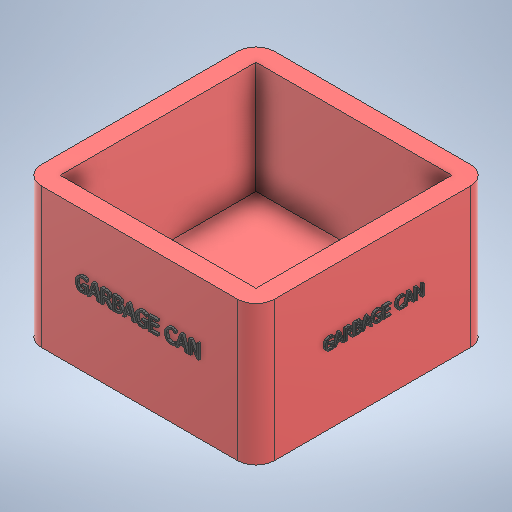
# Autodesk Inventor part: Garbage Can Mockup
Saved by Autodesk Inventor 2025.2 (Build 292293000, 293)
## iProperties
Created: 2025-01-24
Part Number: Garbage Can Mockup
Material: Generic
Document SubType Name: Modeling
Designer: Matt Tidd
Density: 1 g/cm^3
Appearance: Default
Author: Matt Tidd
Autodesk Inventor part; units mm, degrees
ref_plane "YZ Plane" through (0, 0, 0) normal (1, 0, 0) x (0, 1, 0)
ref_plane "XZ Plane" through (0, 0, 0) normal (0, 1, 0) x (-1, 0, 0)
ref_plane "XY Plane" through (0, 0, 0) normal (0, 0, 1) x (1, 0, 0)
sketch "Sketch1" plane through (0, 0, 0) normal (0, 1, 0) x (-1, 0, 0)
  line L0 (0, 0) -> (250, 0)
  line L1 (250, 0) -> (250, -250)
  line L2 (250, -250) -> (0, -250)
  line L3 (0, -250) -> (0, 0)
  dimension "d0" = 250
  dimension "d1" = 250
  constraints: 8 end point, 2 parallel, 1 horizontal, 1 perpendicular
  measures "d0" distance of L1.end L2.end
  measures "d1" distance of L0.end L1.end
extrude "Extrusion1" add sketch "Sketch1" along normal blind 150
fillet "Fillet1" radius 20 4 edges at (0, 75, 0) (-250, 75, 0) (0, 75, -250) (-250, 75, -250)
sketch "Sketch2" plane through (-230, 0, 0) normal (0, 0, 1) x (1, 0, 0)
  line L0 (-20, 0) -> (-20, 150) construction
  line L1 (-20, 75) -> (230, 75) construction
  line L2 (230, 150) -> (230, 0) construction
  spline S0 degree 2 poles (45.9056, 74.7083) (44.3132, 74.7083) (41.6754, 75.6807) (40.7273, 76.6653) knots 0 0 0 1 2 2 2
  spline S1 degree 2 poles (40.7273, 76.6653) (39.7792, 77.6621) (38.7703, 80.6037) (38.7703, 82.5122) knots 0 0 0 1 2 2 2
  spline S2 degree 2 poles (38.7703, 82.5122) (38.7703, 84.3233) (39.7913, 87.1921) (40.7395, 88.2131) knots 0 0 0 1 2 2 2
  spline S3 degree 2 poles (40.7395, 88.2131) (41.6511, 89.1977) (44.3254, 90.2674) (45.9177, 90.2674) knots 0 0 0 1 2 2 2
  spline S4 degree 2 poles (45.9177, 90.2674) (46.6835, 90.2674) (48.0693, 90.0486) (48.7014, 89.8541) knots 0 0 0 1 2 2 2
  spline S5 degree 2 poles (48.7014, 89.8541) (49.2119, 89.7083) (50.4518, 89.1734) (50.8286, 88.9789) knots 0 0 0 1 2 2 2
  line L3 (50.8286, 88.9789) -> (50.8286, 86.5721)
  line L4 (50.8286, 86.5721) -> (50.6584, 86.5721)
  spline S6 degree 2 poles (50.6584, 86.5721) (50.2816, 86.9003) (49.4915, 87.4959) (48.7622, 87.8363) knots 0 0 0 1 2 2 2
  spline S7 degree 2 poles (48.7622, 87.8363) (48.1544, 88.1402) (46.5863, 88.5413) (45.6868, 88.5413) knots 0 0 0 1 2 2 2
  spline S8 degree 2 poles (45.6868, 88.5413) (43.5231, 88.5413) (40.8489, 85.2836) (40.8489, 82.5729) knots 0 0 0 1 2 2 2
  spline S9 degree 2 poles (40.8489, 82.5729) (40.8489, 81.0656) (41.5539, 78.8047) (42.2224, 78.0267) knots 0 0 0 1 2 2 2
  spline S10 degree 2 poles (42.2224, 78.0267) (42.8667, 77.2488) (44.69, 76.4344) (45.8327, 76.4344) knots 0 0 0 1 2 2 2
  spline S11 degree 2 poles (45.8327, 76.4344) (46.6714, 76.4344) (48.3489, 76.6775) (48.9202, 76.9206) knots 0 0 0 1 2 2 2
  line L5 (48.9202, 76.9206) -> (48.9202, 80.7982)
  line L6 (48.9202, 80.7982) -> (45.4437, 80.7982)
  line L7 (45.4437, 80.7982) -> (45.4437, 82.5486)
  line L8 (45.4437, 82.5486) -> (50.8894, 82.5486)
  line L9 (50.8894, 82.5486) -> (50.8894, 75.9968)
  spline S12 degree 2 poles (50.8894, 75.9968) (50.5126, 75.8266) (49.2241, 75.3039) (48.6771, 75.1459) knots 0 0 0 1 2 2 2
  spline S13 degree 2 poles (48.6771, 75.1459) (47.9356, 74.9271) (46.7443, 74.7083) (45.9056, 74.7083) knots 0 0 0 1 2 2 2
  line L10 (51.7767, 75) -> (56.8335, 90)
  line L11 (56.8335, 90) -> (59.2889, 90)
  line L12 (59.2889, 90) -> (64.3456, 75)
  line L13 (64.3456, 75) -> (62.2427, 75)
  line L14 (62.2427, 75) -> (60.8813, 79.1937)
  line L15 (60.8813, 79.1937) -> (55.156, 79.1937)
  line L16 (55.156, 79.1937) -> (53.7946, 75)
  line L17 (53.7946, 75) -> (51.7767, 75)
  line L18 (60.3343, 80.8955) -> (58.0126, 87.9579)
  line L19 (58.0126, 87.9579) -> (55.703, 80.8955)
  line L20 (55.703, 80.8955) -> (60.3343, 80.8955)
  line L21 (77.5709, 75) -> (74.9818, 75)
  line L22 (74.9818, 75) -> (70.2411, 80.9684)
  line L23 (70.2411, 80.9684) -> (67.9558, 80.9684)
  line L24 (67.9558, 80.9684) -> (67.9558, 75)
  line L25 (67.9558, 75) -> (65.9623, 75)
  line L26 (65.9623, 75) -> (65.9623, 90)
  line L27 (65.9623, 90) -> (69.8278, 90)
  spline S14 degree 2 poles (69.8278, 90) (71.1163, 90) (72.8545, 89.7204) (73.6447, 89.2099) knots 0 0 0 1 2 2 2
  spline S15 degree 2 poles (73.6447, 89.2099) (74.4348, 88.6994) (75.3464, 87.107) (75.3464, 85.9279) knots 0 0 0 1 2 2 2
  spline S16 degree 2 poles (75.3464, 85.9279) (75.3464, 84.2869) (73.669, 82.0624) (72.2346, 81.5276) knots 0 0 0 1 2 2 2
  line L28 (72.2346, 81.5276) -> (77.5709, 75)
  spline S17 degree 2 poles (73.2678, 85.7699) (73.2678, 86.4263) (72.8059, 87.4352) (72.3197, 87.7634) knots 0 0 0 1 2 2 2
  spline S18 degree 2 poles (72.3197, 87.7634) (71.8942, 88.0429) (70.7638, 88.2739) (69.9372, 88.2739) knots 0 0 0 1 2 2 2
  line L29 (69.9372, 88.2739) -> (67.9558, 88.2739)
  line L30 (67.9558, 88.2739) -> (67.9558, 82.6337)
  line L31 (67.9558, 82.6337) -> (69.7062, 82.6337)
  spline S19 degree 2 poles (69.7062, 82.6337) (70.5693, 82.6337) (71.9429, 82.9376) (72.4169, 83.4117) knots 0 0 0 1 2 2 2
  spline S20 degree 2 poles (72.4169, 83.4117) (72.8545, 83.825) (73.2678, 84.9919) (73.2678, 85.7699) knots 0 0 0 1 2 2 2
  spline S21 degree 2 poles (88.9364, 79.607) (88.9364, 78.4887) (88.0855, 76.7747) (87.3805, 76.2156) knots 0 0 0 1 2 2 2
  spline S22 degree 2 poles (87.3805, 76.2156) (86.5296, 75.5592) (84.5968, 75) (83.0652, 75) knots 0 0 0 1 2 2 2
  line L32 (83.0652, 75) -> (78.7622, 75)
  line L33 (78.7622, 75) -> (78.7622, 90)
  line L34 (78.7622, 90) -> (82.737, 90)
  spline S23 degree 2 poles (82.737, 90) (84.3416, 90) (85.9461, 89.7934) (86.6754, 89.3922) knots 0 0 0 1 2 2 2
  spline S24 degree 2 poles (86.6754, 89.3922) (87.4899, 88.9668) (88.2314, 87.5689) (88.2314, 86.6207) knots 0 0 0 1 2 2 2
  spline S25 degree 2 poles (88.2314, 86.6207) (88.2314, 85.5632) (87.113, 83.8857) (86.1284, 83.4117) knots 0 0 0 1 2 2 2
  line L35 (86.1284, 83.4117) -> (86.1284, 83.3387)
  spline S26 degree 2 poles (86.1284, 83.3387) (87.4656, 82.9741) (88.9364, 81.0413) (88.9364, 79.607) knots 0 0 0 1 2 2 2
  spline S27 degree 2 poles (86.8578, 79.5219) (86.8578, 80.3728) (86.3716, 81.4668) (85.6422, 81.8558) knots 0 0 0 1 2 2 2
  spline S28 degree 2 poles (85.6422, 81.8558) (85.1682, 82.0989) (84.0498, 82.2447) (83.0166, 82.2447) knots 0 0 0 1 2 2 2
  line L36 (83.0166, 82.2447) -> (80.7557, 82.2447)
  line L37 (80.7557, 82.2447) -> (80.7557, 76.7018)
  line L38 (80.7557, 76.7018) -> (82.3724, 76.7018)
  spline S29 degree 2 poles (82.3724, 76.7018) (83.6852, 76.7018) (85.1925, 76.9449) (85.7759, 77.3339) knots 0 0 0 1 2 2 2
  spline S30 degree 2 poles (85.7759, 77.3339) (86.3351, 77.735) (86.8578, 78.7318) (86.8578, 79.5219) knots 0 0 0 1 2 2 2
  spline S31 degree 2 poles (86.1528, 86.3412) (86.1528, 86.876) (85.7881, 87.6783) (85.387, 87.9092) knots 0 0 0 1 2 2 2
  spline S32 degree 2 poles (85.387, 87.9092) (84.9007, 88.1767) (83.7216, 88.2982) (82.6641, 88.2982) knots 0 0 0 1 2 2 2
  line L39 (82.6641, 88.2982) -> (80.7557, 88.2982)
  line L40 (80.7557, 88.2982) -> (80.7557, 83.91)
  line L41 (80.7557, 83.91) -> (83.0166, 83.91)
  spline S33 degree 2 poles (83.0166, 83.91) (83.9526, 83.91) (84.84, 84.1045) (85.314, 84.4084) knots 0 0 0 1 2 2 2
  spline S34 degree 2 poles (85.314, 84.4084) (85.7759, 84.7002) (86.1528, 85.6361) (86.1528, 86.3412) knots 0 0 0 1 2 2 2
  line L42 (89.3011, 75) -> (94.3578, 90)
  line L43 (94.3578, 90) -> (96.8132, 90)
  line L44 (96.8132, 90) -> (101.8699, 75)
  line L45 (101.8699, 75) -> (99.767, 75)
  line L46 (99.767, 75) -> (98.4056, 79.1937)
  line L47 (98.4056, 79.1937) -> (92.6803, 79.1937)
  line L48 (92.6803, 79.1937) -> (91.3189, 75)
  line L49 (91.3189, 75) -> (89.3011, 75)
  line L50 (97.8586, 80.8955) -> (95.5369, 87.9579)
  line L51 (95.5369, 87.9579) -> (93.2273, 80.8955)
  line L52 (93.2273, 80.8955) -> (97.8586, 80.8955)
  spline S35 degree 2 poles (109.7711, 74.7083) (108.1787, 74.7083) (105.5409, 75.6807) (104.5928, 76.6653) knots 0 0 0 1 2 2 2
  spline S36 degree 2 poles (104.5928, 76.6653) (103.6447, 77.6621) (102.6357, 80.6037) (102.6357, 82.5122) knots 0 0 0 1 2 2 2
  spline S37 degree 2 poles (102.6357, 82.5122) (102.6357, 84.3233) (103.6568, 87.1921) (104.6049, 88.2131) knots 0 0 0 1 2 2 2
  spline S38 degree 2 poles (104.6049, 88.2131) (105.5166, 89.1977) (108.1908, 90.2674) (109.7832, 90.2674) knots 0 0 0 1 2 2 2
  spline S39 degree 2 poles (109.7832, 90.2674) (110.549, 90.2674) (111.9348, 90.0486) (112.5669, 89.8541) knots 0 0 0 1 2 2 2
  spline S40 degree 2 poles (112.5669, 89.8541) (113.0774, 89.7083) (114.3173, 89.1734) (114.6941, 88.9789) knots 0 0 0 1 2 2 2
  line L53 (114.6941, 88.9789) -> (114.6941, 86.5721)
  line L54 (114.6941, 86.5721) -> (114.5239, 86.5721)
  spline S41 degree 2 poles (114.5239, 86.5721) (114.1471, 86.9003) (113.357, 87.4959) (112.6276, 87.8363) knots 0 0 0 1 2 2 2
  spline S42 degree 2 poles (112.6276, 87.8363) (112.0199, 88.1402) (110.4518, 88.5413) (109.5523, 88.5413) knots 0 0 0 1 2 2 2
  spline S43 degree 2 poles (109.5523, 88.5413) (107.3886, 88.5413) (104.7143, 85.2836) (104.7143, 82.5729) knots 0 0 0 1 2 2 2
  spline S44 degree 2 poles (104.7143, 82.5729) (104.7143, 81.0656) (105.4194, 78.8047) (106.0879, 78.0267) knots 0 0 0 1 2 2 2
  spline S45 degree 2 poles (106.0879, 78.0267) (106.7322, 77.2488) (108.5555, 76.4344) (109.6981, 76.4344) knots 0 0 0 1 2 2 2
  spline S46 degree 2 poles (109.6981, 76.4344) (110.5369, 76.4344) (112.2143, 76.6775) (112.7857, 76.9206) knots 0 0 0 1 2 2 2
  line L55 (112.7857, 76.9206) -> (112.7857, 80.7982)
  line L56 (112.7857, 80.7982) -> (109.3092, 80.7982)
  line L57 (109.3092, 80.7982) -> (109.3092, 82.5486)
  line L58 (109.3092, 82.5486) -> (114.7549, 82.5486)
  line L59 (114.7549, 82.5486) -> (114.7549, 75.9968)
  spline S47 degree 2 poles (114.7549, 75.9968) (114.378, 75.8266) (113.0895, 75.3039) (112.5425, 75.1459) knots 0 0 0 1 2 2 2
  spline S48 degree 2 poles (112.5425, 75.1459) (111.8011, 74.9271) (110.6098, 74.7083) (109.7711, 74.7083) knots 0 0 0 1 2 2 2
  line L60 (117.2589, 75) -> (117.2589, 90)
  line L61 (117.2589, 90) -> (126.643, 90)
  line L62 (126.643, 90) -> (126.643, 88.2253)
  line L63 (126.643, 88.2253) -> (119.2524, 88.2253)
  line L64 (119.2524, 88.2253) -> (119.2524, 84.1167)
  line L65 (119.2524, 84.1167) -> (126.1447, 84.1167)
  line L66 (126.1447, 84.1167) -> (126.1447, 82.342)
  line L67 (126.1447, 82.342) -> (119.2524, 82.342)
  line L68 (119.2524, 82.342) -> (119.2524, 76.7747)
  line L69 (119.2524, 76.7747) -> (126.643, 76.7747)
  line L70 (126.643, 76.7747) -> (126.643, 75)
  line L71 (126.643, 75) -> (117.2589, 75)
  spline S49 degree 2 poles (141.1325, 74.7326) (139.6738, 74.7326) (137.2062, 75.7172) (136.3067, 76.7018) knots 0 0 0 1 2 2 2
  spline S50 degree 2 poles (136.3067, 76.7018) (135.4072, 77.6742) (134.4226, 80.5916) (134.4226, 82.4878) knots 0 0 0 1 2 2 2
  spline S51 degree 2 poles (134.4226, 82.4878) (134.4226, 84.372) (135.3829, 87.1677) (136.2946, 88.201) knots 0 0 0 1 2 2 2
  spline S52 degree 2 poles (136.2946, 88.201) (137.1941, 89.2099) (139.6495, 90.2674) (141.169, 90.2674) knots 0 0 0 1 2 2 2
  spline S53 degree 2 poles (141.169, 90.2674) (141.9226, 90.2674) (143.2476, 90.0486) (143.8067, 89.8784) knots 0 0 0 1 2 2 2
  spline S54 degree 2 poles (143.8067, 89.8784) (144.293, 89.7204) (145.3019, 89.2707) (145.8002, 89.0032) knots 0 0 0 1 2 2 2
  line L72 (145.8002, 89.0032) -> (145.8002, 86.5964)
  line L73 (145.8002, 86.5964) -> (145.6422, 86.5964)
  spline S55 degree 2 poles (145.6422, 86.5964) (145.3748, 86.8395) (144.5482, 87.5203) (143.9526, 87.8485) knots 0 0 0 1 2 2 2
  spline S56 degree 2 poles (143.9526, 87.8485) (143.3813, 88.1645) (142.032, 88.5656) (141.1568, 88.5656) knots 0 0 0 1 2 2 2
  spline S57 degree 2 poles (141.1568, 88.5656) (140.1965, 88.5656) (138.4826, 87.7755) (137.8383, 87.0219) knots 0 0 0 1 2 2 2
  spline S58 degree 2 poles (137.8383, 87.0219) (137.2062, 86.2561) (136.5012, 83.9344) (136.5012, 82.4878) knots 0 0 0 1 2 2 2
  spline S59 degree 2 poles (136.5012, 82.4878) (136.5012, 80.9441) (137.2427, 78.7196) (137.887, 77.9538) knots 0 0 0 1 2 2 2
  spline S60 degree 2 poles (137.887, 77.9538) (138.519, 77.2123) (140.2087, 76.4587) (141.1568, 76.4587) knots 0 0 0 1 2 2 2
  spline S61 degree 2 poles (141.1568, 76.4587) (142.0199, 76.4587) (143.4907, 76.8841) (144.062, 77.2002) knots 0 0 0 1 2 2 2
  spline S62 degree 2 poles (144.062, 77.2002) (144.609, 77.5162) (145.4234, 78.1726) (145.6544, 78.4036) knots 0 0 0 1 2 2 2
  line L74 (145.6544, 78.4036) -> (145.8002, 78.4036)
  line L75 (145.8002, 78.4036) -> (145.8002, 76.0211)
  spline S63 degree 2 poles (145.8002, 76.0211) (145.3019, 75.7901) (144.4267, 75.3647) (143.8067, 75.1702) knots 0 0 0 1 2 2 2
  spline S64 degree 2 poles (143.8067, 75.1702) (143.1503, 74.9514) (142.032, 74.7326) (141.1325, 74.7326) knots 0 0 0 1 2 2 2
  line L76 (146.0434, 75) -> (151.1001, 90)
  line L77 (151.1001, 90) -> (153.5555, 90)
  line L78 (153.5555, 90) -> (158.6122, 75)
  line L79 (158.6122, 75) -> (156.5093, 75)
  line L80 (156.5093, 75) -> (155.1479, 79.1937)
  line L81 (155.1479, 79.1937) -> (149.4226, 79.1937)
  line L82 (149.4226, 79.1937) -> (148.0612, 75)
  line L83 (148.0612, 75) -> (146.0434, 75)
  line L84 (154.6009, 80.8955) -> (152.2792, 87.9579)
  line L85 (152.2792, 87.9579) -> (149.9696, 80.8955)
  line L86 (149.9696, 80.8955) -> (154.6009, 80.8955)
  line L87 (170.9623, 75) -> (168.7257, 75)
  line L88 (168.7257, 75) -> (162.0887, 87.9335)
  line L89 (162.0887, 87.9335) -> (162.0887, 75)
  line L90 (162.0887, 75) -> (160.2289, 75)
  line L91 (160.2289, 75) -> (160.2289, 90)
  line L92 (160.2289, 90) -> (163.0612, 90)
  line L93 (163.0612, 90) -> (169.1025, 78.124)
  line L94 (169.1025, 78.124) -> (169.1025, 90)
  line L95 (169.1025, 90) -> (170.9623, 90)
  line L96 (170.9623, 90) -> (170.9623, 75)
  constraints: 2 end point, 2 midpoint, 1 horizontal
extrude "Extrusion2" add sketch "Sketch2" along normal blind 2.5
sketch "Sketch3" plane through (0, 150, 0) normal (0, 1, 0) x (1, 0, 0)
  line L0 (-250, 230) -> (-250, 20) construction
  line L1 (-250, 125) -> (0, 125) construction
  line L2 (0, 20) -> (0, 230) construction
  line L3 (-230, 0) -> (-20, 0) construction
  line L4 (-125, 0) -> (-125, 250) construction
  line L5 (-20, 250) -> (-230, 250) construction
  point P0 (0, 0)
  point P1 (-125, 125)
  constraints: 5 midpoint, 4 end point
pattern_circular "Circular Pattern1" count 2 over 360 about axis through (-125, 150, -125) along (0, 1, 0) of "Extrusion2"
sketch "Sketch4" plane through (0, 0, -20) normal (1, 0, 0) x (0, 0, -1)
  line L0 (-20, 0) -> (-20, 150) construction
  line L1 (-20, 75) -> (230, 75) construction
  line L2 (230, 150) -> (230, 0) construction
  spline S0 degree 2 poles (57.7245, 74.7666) (56.4506, 74.7666) (54.3404, 75.5446) (53.5818, 76.3323) knots 0 0 0 1 2 2 2
  spline S1 degree 2 poles (53.5818, 76.3323) (52.8233, 77.1297) (52.0162, 79.483) (52.0162, 81.0097) knots 0 0 0 1 2 2 2
  spline S2 degree 2 poles (52.0162, 81.0097) (52.0162, 82.4587) (52.8331, 84.7536) (53.5916, 85.5705) knots 0 0 0 1 2 2 2
  spline S3 degree 2 poles (53.5916, 85.5705) (54.3209, 86.3582) (56.4603, 87.2139) (57.7342, 87.2139) knots 0 0 0 1 2 2 2
  spline S4 degree 2 poles (57.7342, 87.2139) (58.3468, 87.2139) (59.4554, 87.0389) (59.9611, 86.8833) knots 0 0 0 1 2 2 2
  spline S5 degree 2 poles (59.9611, 86.8833) (60.3695, 86.7666) (61.3614, 86.3387) (61.6629, 86.1831) knots 0 0 0 1 2 2 2
  line L3 (61.6629, 86.1831) -> (61.6629, 84.2577)
  line L4 (61.6629, 84.2577) -> (61.5267, 84.2577)
  spline S6 degree 2 poles (61.5267, 84.2577) (61.2253, 84.5203) (60.5932, 84.9968) (60.0097, 85.269) knots 0 0 0 1 2 2 2
  spline S7 degree 2 poles (60.0097, 85.269) (59.5235, 85.5122) (58.269, 85.8331) (57.5494, 85.8331) knots 0 0 0 1 2 2 2
  spline S8 degree 2 poles (57.5494, 85.8331) (55.8185, 85.8331) (53.6791, 83.2269) (53.6791, 81.0583) knots 0 0 0 1 2 2 2
  spline S9 degree 2 poles (53.6791, 81.0583) (53.6791, 79.8525) (54.2431, 78.0438) (54.778, 77.4214) knots 0 0 0 1 2 2 2
  spline S10 degree 2 poles (54.778, 77.4214) (55.2934, 76.799) (56.752, 76.1475) (57.6661, 76.1475) knots 0 0 0 1 2 2 2
  spline S11 degree 2 poles (57.6661, 76.1475) (58.3371, 76.1475) (59.6791, 76.342) (60.1361, 76.5365) knots 0 0 0 1 2 2 2
  line L5 (60.1361, 76.5365) -> (60.1361, 79.6386)
  line L6 (60.1361, 79.6386) -> (57.3549, 79.6386)
  line L7 (57.3549, 79.6386) -> (57.3549, 81.0389)
  line L8 (57.3549, 81.0389) -> (61.7115, 81.0389)
  line L9 (61.7115, 81.0389) -> (61.7115, 75.7974)
  spline S12 degree 2 poles (61.7115, 75.7974) (61.41, 75.6613) (60.3793, 75.2431) (59.9416, 75.1167) knots 0 0 0 1 2 2 2
  spline S13 degree 2 poles (59.9416, 75.1167) (59.3485, 74.9417) (58.3955, 74.7666) (57.7245, 74.7666) knots 0 0 0 1 2 2 2
  line L10 (62.4214, 75) -> (66.4668, 87)
  line L11 (66.4668, 87) -> (68.4311, 87)
  line L12 (68.4311, 87) -> (72.4765, 75)
  line L13 (72.4765, 75) -> (70.7942, 75)
  line L14 (70.7942, 75) -> (69.705, 78.3549)
  line L15 (69.705, 78.3549) -> (65.1248, 78.3549)
  line L16 (65.1248, 78.3549) -> (64.0357, 75)
  line L17 (64.0357, 75) -> (62.4214, 75)
  line L18 (69.2674, 79.7164) -> (67.41, 85.3663)
  line L19 (67.41, 85.3663) -> (65.5624, 79.7164)
  line L20 (65.5624, 79.7164) -> (69.2674, 79.7164)
  line L21 (83.0567, 75) -> (80.9854, 75)
  line L22 (80.9854, 75) -> (77.1929, 79.7747)
  line L23 (77.1929, 79.7747) -> (75.3647, 79.7747)
  line L24 (75.3647, 79.7747) -> (75.3647, 75)
  line L25 (75.3647, 75) -> (73.7699, 75)
  line L26 (73.7699, 75) -> (73.7699, 87)
  line L27 (73.7699, 87) -> (76.8622, 87)
  spline S14 degree 2 poles (76.8622, 87) (77.893, 87) (79.2836, 86.7763) (79.9157, 86.3679) knots 0 0 0 1 2 2 2
  spline S15 degree 2 poles (79.9157, 86.3679) (80.5478, 85.9595) (81.2771, 84.6856) (81.2771, 83.7423) knots 0 0 0 1 2 2 2
  spline S16 degree 2 poles (81.2771, 83.7423) (81.2771, 82.4295) (79.9352, 80.6499) (78.7877, 80.222) knots 0 0 0 1 2 2 2
  line L28 (78.7877, 80.222) -> (83.0567, 75)
  spline S17 degree 2 poles (79.6143, 83.6159) (79.6143, 84.141) (79.2447, 84.9481) (78.8558, 85.2107) knots 0 0 0 1 2 2 2
  spline S18 degree 2 poles (78.8558, 85.2107) (78.5154, 85.4344) (77.611, 85.6191) (76.9498, 85.6191) knots 0 0 0 1 2 2 2
  line L29 (76.9498, 85.6191) -> (75.3647, 85.6191)
  line L30 (75.3647, 85.6191) -> (75.3647, 81.107)
  line L31 (75.3647, 81.107) -> (76.765, 81.107)
  spline S19 degree 2 poles (76.765, 81.107) (77.4554, 81.107) (78.5543, 81.3501) (78.9335, 81.7293) knots 0 0 0 1 2 2 2
  spline S20 degree 2 poles (78.9335, 81.7293) (79.2836, 82.06) (79.6143, 82.9935) (79.6143, 83.6159) knots 0 0 0 1 2 2 2
  spline S21 degree 2 poles (92.1491, 78.6856) (92.1491, 77.7909) (91.4684, 76.4198) (90.9044, 75.9724) knots 0 0 0 1 2 2 2
  spline S22 degree 2 poles (90.9044, 75.9724) (90.2237, 75.4473) (88.6775, 75) (87.4522, 75) knots 0 0 0 1 2 2 2
  line L32 (87.4522, 75) -> (84.0097, 75)
  line L33 (84.0097, 75) -> (84.0097, 87)
  line L34 (84.0097, 87) -> (87.1896, 87)
  spline S23 degree 2 poles (87.1896, 87) (88.4733, 87) (89.7569, 86.8347) (90.3404, 86.5138) knots 0 0 0 1 2 2 2
  spline S24 degree 2 poles (90.3404, 86.5138) (90.9919, 86.1734) (91.5851, 85.0551) (91.5851, 84.2966) knots 0 0 0 1 2 2 2
  spline S25 degree 2 poles (91.5851, 84.2966) (91.5851, 83.4506) (90.6904, 82.1086) (89.9028, 81.7293) knots 0 0 0 1 2 2 2
  line L35 (89.9028, 81.7293) -> (89.9028, 81.671)
  spline S26 degree 2 poles (89.9028, 81.671) (90.9724, 81.3793) (92.1491, 79.8331) (92.1491, 78.6856) knots 0 0 0 1 2 2 2
  spline S27 degree 2 poles (90.4862, 78.6175) (90.4862, 79.2982) (90.0972, 80.1734) (89.5138, 80.4846) knots 0 0 0 1 2 2 2
  spline S28 degree 2 poles (89.5138, 80.4846) (89.1345, 80.6791) (88.2399, 80.7958) (87.4133, 80.7958) knots 0 0 0 1 2 2 2
  line L36 (87.4133, 80.7958) -> (85.6045, 80.7958)
  line L37 (85.6045, 80.7958) -> (85.6045, 76.3614)
  line L38 (85.6045, 76.3614) -> (86.8979, 76.3614)
  spline S29 degree 2 poles (86.8979, 76.3614) (87.9481, 76.3614) (89.154, 76.5559) (89.6207, 76.8671) knots 0 0 0 1 2 2 2
  spline S30 degree 2 poles (89.6207, 76.8671) (90.0681, 77.188) (90.4862, 77.9854) (90.4862, 78.6175) knots 0 0 0 1 2 2 2
  spline S31 degree 2 poles (89.9222, 84.0729) (89.9222, 84.5008) (89.6305, 85.1426) (89.3096, 85.3274) knots 0 0 0 1 2 2 2
  spline S32 degree 2 poles (89.3096, 85.3274) (88.9206, 85.5413) (87.9773, 85.6386) (87.1313, 85.6386) knots 0 0 0 1 2 2 2
  line L39 (87.1313, 85.6386) -> (85.6045, 85.6386)
  line L40 (85.6045, 85.6386) -> (85.6045, 82.128)
  line L41 (85.6045, 82.128) -> (87.4133, 82.128)
  spline S33 degree 2 poles (87.4133, 82.128) (88.1621, 82.128) (88.872, 82.2836) (89.2512, 82.5267) knots 0 0 0 1 2 2 2
  spline S34 degree 2 poles (89.2512, 82.5267) (89.6207, 82.7601) (89.9222, 83.5089) (89.9222, 84.0729) knots 0 0 0 1 2 2 2
  line L42 (92.4408, 75) -> (96.4862, 87)
  line L43 (96.4862, 87) -> (98.4506, 87)
  line L44 (98.4506, 87) -> (102.4959, 75)
  line L45 (102.4959, 75) -> (100.8136, 75)
  line L46 (100.8136, 75) -> (99.7245, 78.3549)
  line L47 (99.7245, 78.3549) -> (95.1442, 78.3549)
  line L48 (95.1442, 78.3549) -> (94.0551, 75)
  line L49 (94.0551, 75) -> (92.4408, 75)
  line L50 (99.2869, 79.7164) -> (97.4295, 85.3663)
  line L51 (97.4295, 85.3663) -> (95.5818, 79.7164)
  line L52 (95.5818, 79.7164) -> (99.2869, 79.7164)
  spline S35 degree 2 poles (108.8169, 74.7666) (107.5429, 74.7666) (105.4327, 75.5446) (104.6742, 76.3323) knots 0 0 0 1 2 2 2
  spline S36 degree 2 poles (104.6742, 76.3323) (103.9157, 77.1297) (103.1086, 79.483) (103.1086, 81.0097) knots 0 0 0 1 2 2 2
  spline S37 degree 2 poles (103.1086, 81.0097) (103.1086, 82.4587) (103.9254, 84.7536) (104.684, 85.5705) knots 0 0 0 1 2 2 2
  spline S38 degree 2 poles (104.684, 85.5705) (105.4133, 86.3582) (107.5527, 87.2139) (108.8266, 87.2139) knots 0 0 0 1 2 2 2
  spline S39 degree 2 poles (108.8266, 87.2139) (109.4392, 87.2139) (110.5478, 87.0389) (111.0535, 86.8833) knots 0 0 0 1 2 2 2
  spline S40 degree 2 poles (111.0535, 86.8833) (111.4619, 86.7666) (112.4538, 86.3387) (112.7553, 86.1831) knots 0 0 0 1 2 2 2
  line L53 (112.7553, 86.1831) -> (112.7553, 84.2577)
  line L54 (112.7553, 84.2577) -> (112.6191, 84.2577)
  spline S41 degree 2 poles (112.6191, 84.2577) (112.3177, 84.5203) (111.6856, 84.9968) (111.1021, 85.269) knots 0 0 0 1 2 2 2
  spline S42 degree 2 poles (111.1021, 85.269) (110.6159, 85.5122) (109.3614, 85.8331) (108.6418, 85.8331) knots 0 0 0 1 2 2 2
  spline S43 degree 2 poles (108.6418, 85.8331) (106.9109, 85.8331) (104.7715, 83.2269) (104.7715, 81.0583) knots 0 0 0 1 2 2 2
  spline S44 degree 2 poles (104.7715, 81.0583) (104.7715, 79.8525) (105.3355, 78.0438) (105.8703, 77.4214) knots 0 0 0 1 2 2 2
  spline S45 degree 2 poles (105.8703, 77.4214) (106.3857, 76.799) (107.8444, 76.1475) (108.7585, 76.1475) knots 0 0 0 1 2 2 2
  spline S46 degree 2 poles (108.7585, 76.1475) (109.4295, 76.1475) (110.7715, 76.342) (111.2285, 76.5365) knots 0 0 0 1 2 2 2
  line L55 (111.2285, 76.5365) -> (111.2285, 79.6386)
  line L56 (111.2285, 79.6386) -> (108.4473, 79.6386)
  line L57 (108.4473, 79.6386) -> (108.4473, 81.0389)
  line L58 (108.4473, 81.0389) -> (112.8039, 81.0389)
  line L59 (112.8039, 81.0389) -> (112.8039, 75.7974)
  spline S47 degree 2 poles (112.8039, 75.7974) (112.5024, 75.6613) (111.4716, 75.2431) (111.034, 75.1167) knots 0 0 0 1 2 2 2
  spline S48 degree 2 poles (111.034, 75.1167) (110.4408, 74.9417) (109.4878, 74.7666) (108.8169, 74.7666) knots 0 0 0 1 2 2 2
  line L60 (114.8071, 75) -> (114.8071, 87)
  line L61 (114.8071, 87) -> (122.3144, 87)
  line L62 (122.3144, 87) -> (122.3144, 85.5802)
  line L63 (122.3144, 85.5802) -> (116.4019, 85.5802)
  line L64 (116.4019, 85.5802) -> (116.4019, 82.2934)
  line L65 (116.4019, 82.2934) -> (121.9157, 82.2934)
  line L66 (121.9157, 82.2934) -> (121.9157, 80.8736)
  line L67 (121.9157, 80.8736) -> (116.4019, 80.8736)
  line L68 (116.4019, 80.8736) -> (116.4019, 76.4198)
  line L69 (116.4019, 76.4198) -> (122.3144, 76.4198)
  line L70 (122.3144, 76.4198) -> (122.3144, 75)
  line L71 (122.3144, 75) -> (114.8071, 75)
  spline S49 degree 2 poles (133.906, 74.7861) (132.7391, 74.7861) (130.765, 75.5737) (130.0454, 76.3614) knots 0 0 0 1 2 2 2
  spline S50 degree 2 poles (130.0454, 76.3614) (129.3258, 77.1394) (128.5381, 79.4733) (128.5381, 80.9903) knots 0 0 0 1 2 2 2
  spline S51 degree 2 poles (128.5381, 80.9903) (128.5381, 82.4976) (129.3063, 84.7342) (130.0357, 85.5608) knots 0 0 0 1 2 2 2
  spline S52 degree 2 poles (130.0357, 85.5608) (130.7553, 86.3679) (132.7196, 87.2139) (133.9352, 87.2139) knots 0 0 0 1 2 2 2
  spline S53 degree 2 poles (133.9352, 87.2139) (134.5381, 87.2139) (135.5981, 87.0389) (136.0454, 86.9028) knots 0 0 0 1 2 2 2
  spline S54 degree 2 poles (136.0454, 86.9028) (136.4344, 86.7763) (137.2415, 86.4165) (137.6402, 86.2026) knots 0 0 0 1 2 2 2
  line L72 (137.6402, 86.2026) -> (137.6402, 84.2771)
  line L73 (137.6402, 84.2771) -> (137.5138, 84.2771)
  spline S55 degree 2 poles (137.5138, 84.2771) (137.2998, 84.4716) (136.6386, 85.0162) (136.1621, 85.2788) knots 0 0 0 1 2 2 2
  spline S56 degree 2 poles (136.1621, 85.2788) (135.705, 85.5316) (134.6256, 85.8525) (133.9254, 85.8525) knots 0 0 0 1 2 2 2
  spline S57 degree 2 poles (133.9254, 85.8525) (133.1572, 85.8525) (131.7861, 85.2204) (131.2707, 84.6175) knots 0 0 0 1 2 2 2
  spline S58 degree 2 poles (131.2707, 84.6175) (130.765, 84.0049) (130.201, 82.1475) (130.201, 80.9903) knots 0 0 0 1 2 2 2
  spline S59 degree 2 poles (130.201, 80.9903) (130.201, 79.7553) (130.7942, 77.9757) (131.3096, 77.363) knots 0 0 0 1 2 2 2
  spline S60 degree 2 poles (131.3096, 77.363) (131.8152, 76.7699) (133.1669, 76.1669) (133.9254, 76.1669) knots 0 0 0 1 2 2 2
  spline S61 degree 2 poles (133.9254, 76.1669) (134.6159, 76.1669) (135.7925, 76.5073) (136.2496, 76.7601) knots 0 0 0 1 2 2 2
  spline S62 degree 2 poles (136.2496, 76.7601) (136.6872, 77.013) (137.3387, 77.5381) (137.5235, 77.7229) knots 0 0 0 1 2 2 2
  line L74 (137.5235, 77.7229) -> (137.6402, 77.7229)
  line L75 (137.6402, 77.7229) -> (137.6402, 75.8169)
  spline S63 degree 2 poles (137.6402, 75.8169) (137.2415, 75.6321) (136.5413, 75.2917) (136.0454, 75.1361) knots 0 0 0 1 2 2 2
  spline S64 degree 2 poles (136.0454, 75.1361) (135.5203, 74.9611) (134.6256, 74.7861) (133.906, 74.7861) knots 0 0 0 1 2 2 2
  line L76 (137.8347, 75) -> (141.8801, 87)
  line L77 (141.8801, 87) -> (143.8444, 87)
  line L78 (143.8444, 87) -> (147.8898, 75)
  line L79 (147.8898, 75) -> (146.2075, 75)
  line L80 (146.2075, 75) -> (145.1183, 78.3549)
  line L81 (145.1183, 78.3549) -> (140.5381, 78.3549)
  line L82 (140.5381, 78.3549) -> (139.4489, 75)
  line L83 (139.4489, 75) -> (137.8347, 75)
  line L84 (144.6807, 79.7164) -> (142.8233, 85.3663)
  line L85 (142.8233, 85.3663) -> (140.9757, 79.7164)
  line L86 (140.9757, 79.7164) -> (144.6807, 79.7164)
  line L87 (157.7699, 75) -> (155.9806, 75)
  line L88 (155.9806, 75) -> (150.671, 85.3468)
  line L89 (150.671, 85.3468) -> (150.671, 75)
  line L90 (150.671, 75) -> (149.1831, 75)
  line L91 (149.1831, 75) -> (149.1831, 87)
  line L92 (149.1831, 87) -> (151.4489, 87)
  line L93 (151.4489, 87) -> (156.282, 77.4992)
  line L94 (156.282, 77.4992) -> (156.282, 87)
  line L95 (156.282, 87) -> (157.7699, 87)
  line L96 (157.7699, 87) -> (157.7699, 75)
  constraints: 2 end point, 2 midpoint, 1 horizontal
extrude "Extrusion3" add sketch "Sketch4" along normal blind 2.5
pattern_circular "Circular Pattern2" count 2 over 360 about axis through (-125, 150, -125) along (0, 1, 0) of "Extrusion3"
sketch "Sketch5" plane through (0, 150, 0) normal (0, 1, 0) x (1, 0, 0)
  arc A0 (-230, 250) -> (-250, 230) centre (-230, 230) ccw projected
  line L0 (-250, 230) -> (-250, 20) projected
  arc A1 (-250, 20) -> (-230, 0) centre (-230, 20) ccw projected
  line L1 (-230, 0) -> (-20, 0) projected
  arc A2 (-20, 0) -> (0, 20) centre (-20, 20) ccw projected
  line L2 (0, 20) -> (0, 230) projected
  arc A3 (0, 230) -> (-20, 250) centre (-20, 230) ccw projected
  line L3 (-20, 250) -> (-230, 250) projected
  line L4 (-230, 230) -> (-20, 230)
  line L5 (-20, 230) -> (-20, 20)
  line L6 (-20, 20) -> (-230, 20)
  line L7 (-230, 20) -> (-230, 230)
  point P0 (0, 0)
  constraints: 8 end point, 3 other
extrude "Extrusion4" cut sketch "Sketch5" against normal blind 120 contours L4 L5 L6 L7
body "Solid1"
